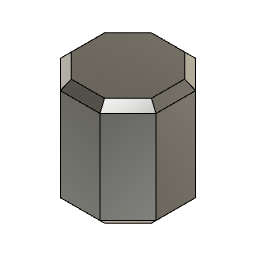
Wobble_Pin v8 (Autodesk Fusion 360 design; units mm, degrees)
Autodesk Fusion 360 part; units mm, degrees
sketch "Sketch1" plane through (0, 0, 0) normal (0, 0, 1) x (1, 0, 0)
  circle A0 centre (0, 0) radius 3.35 construction
  line L0 (1.282, 3.095) -> (-1.282, 3.095)
  line L1 (-1.282, 3.095) -> (-3.095, 1.282)
  line L2 (-3.095, 1.282) -> (-3.095, -1.282)
  line L3 (-3.095, -1.282) -> (-1.282, -3.095)
  line L4 (-1.282, -3.095) -> (1.282, -3.095)
  line L5 (1.282, -3.095) -> (3.095, -1.282)
  line L6 (3.095, -1.282) -> (3.095, 1.282)
  line L7 (3.095, 1.282) -> (1.282, 3.095)
  dimension "d1" = 6.7
  constraint coincident A0.centre origin
  constraint coincident A0 L0.start
  constraint horizontal L0
  measures "d1" diameter of A0
extrude "Extrude1" add sketch "Sketch1" along normal blind 7
chamfer "Chamfer1" distance 0.5 angle 45 8 edges at (-2.1885, 2.1885, 7) (-3.095, 0, 7) (-2.1885, -2.1885, 7) (2.1885, -2.1885, 7) (3.095, 0, 7) (2.1885, 2.1885, 7) (0, 3.095, 7) (0, -3.095, 7)
chamfer "Chamfer2" distance 0.5 angle 45 8 edges at (2.1885, -2.1885, 0) (-2.1885, -2.1885, 0) (-3.095, 0, 0) (-2.1885, 2.1885, 0) (0, 3.095, 0) (2.1885, 2.1885, 0) (3.095, 0, 0) (0, -3.095, 0)
